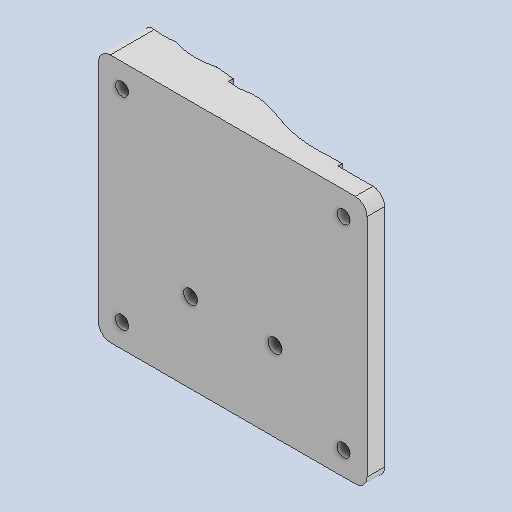
# Autodesk Inventor part: mouldingPlate_V6
Saved by Autodesk Inventor 2023 (Build 270158000, 158)
## iProperties
Created: 2023-03-15
Part Number: mouldingPlate_V6
Material: Generic
Document SubType Name: Modeling
Designer: shrey
Density: 1 g/cm^3
Appearance: Default
Author: shrey
Autodesk Inventor part; units mm, degrees
ref_plane "YZ Plane" through (0, 0, 0) normal (1, 0, 0) x (0, 1, 0)
ref_plane "XZ Plane" through (0, 0, 0) normal (0, 1, 0) x (-1, 0, 0)
ref_plane "XY Plane" through (0, 0, 0) normal (0, 0, 1) x (1, 0, 0)
ref_plane "Work Plane1" through (-64.2812, 0, 0) normal (0, 0, -1) x (1, 0, 0)
sketch "Sketch1" plane through (-64.2812, 0, 0) normal (0, 0, -1) x (1, 0, 0)
  line L0 (64.2812, -304.8) -> (64.2812, 304.8) construction
  line L1 (64.2812, -304.8) -> (0, -304.8) construction
  line L2 (6.11, 304.8) -> (0, 304.8) construction
  line L3 (0, -304.8) -> (6.11, -304.8) construction
  line L4 (6.2392, -19.8934) -> (64.0072, -19.8934) construction
  line L5 (64.0072, -19.8934) -> (64.0072, -14.3934) construction
  line L6 (64.0072, -14.3934) -> (6.2392, -14.3934) construction
  line L7 (6.2392, -14.3934) -> (6.2392, -19.8934) construction
  spline S0 degree 3 poles (60.7862, -9) (60.9061, -9.1901) (61.0858, -9.4753) (61.3069, -9.8666) (61.4657, -10.1639) (61.6162, -10.4656) (61.7579, -10.7714) (61.8899, -11.0816) (62.0114, -11.3961) (62.1204, -11.7151) (62.2163, -12.0383) (62.2788, -12.3122) (62.3239, -12.5324) (62.3716, -12.6943) (62.436, -12.8503) (62.5199, -12.997) (62.6084, -13.1066) (62.6883, -13.1859) (62.7558, -13.2363) (62.8251, -13.2847) (62.9013, -13.3209) (62.9789, -13.3544) (63.0609, -13.3742) (63.1437, -13.3909) (63.2562, -13.3949) (63.3966, -13.3923) (63.5369, -13.3949) (63.6495, -13.3909) (63.7322, -13.3742) (63.8143, -13.3544) (63.8918, -13.3209) (63.9681, -13.2847) (64.0373, -13.2363) (64.1049, -13.1859) (64.1848, -13.1066) (64.2733, -12.997) (64.3572, -12.8503) (64.4216, -12.6943) (64.4693, -12.5324) (64.5144, -12.3122) (64.5768, -12.0383) (64.6728, -11.7151) (64.7818, -11.3961) (64.9032, -11.0816) (65.0353, -10.7714) (65.177, -10.4656) (65.3275, -10.1639) (65.4863, -9.8666) (65.7074, -9.4753) (65.8871, -9.1901) (66.007, -9) knots 0 0 0 0 0.067405 0.101109 0.134814 0.168518 0.202222 0.235926 0.26963 0.303333 0.337035 0.370735 0.387584 0.40443 0.421277 0.438116 0.454951 0.463377 0.471802 0.480225 0.488651 0.497074 0.505499 0.513923 0.522347 0.5392 0.556053 0.564477 0.572901 0.581327 0.589749 0.598176 0.606598 0.615023 0.623449 0.640284 0.657123 0.67397 0.690816 0.707665 0.741365 0.775067 0.80877 0.842474 0.876178 0.909882 0.943586 0.977291 1.010995 1.0784 1.0784 1.0784 1.0784 construction
  line L8 (66.0072, -9) -> (66.007, -9) construction
  line L9 (66.0072, -20.8934) -> (66.0072, -9) construction
  line L10 (4.2392, -20.8934) -> (66.0072, -20.8934) construction
  line L11 (4.2392, -9) -> (4.2392, -20.8934) construction
  spline S1 degree 3 poles (4.2392, -9) (4.3591, -9.1901) (4.5388, -9.4753) (4.7599, -9.8666) (4.9187, -10.1639) (5.0692, -10.4656) (5.2109, -10.7714) (5.3429, -11.0816) (5.4644, -11.3961) (5.5734, -11.7151) (5.6693, -12.0383) (5.7318, -12.3122) (5.7769, -12.5324) (5.8246, -12.6943) (5.889, -12.8503) (5.9729, -12.997) (6.0614, -13.1066) (6.1413, -13.1859) (6.2088, -13.2363) (6.2781, -13.2847) (6.3543, -13.3209) (6.4319, -13.3544) (6.5139, -13.3742) (6.5967, -13.3909) (6.7092, -13.3949) (6.8496, -13.3923) (6.9899, -13.3949) (7.1025, -13.3909) (7.1852, -13.3742) (7.2673, -13.3544) (7.3448, -13.3209) (7.4211, -13.2847) (7.4903, -13.2363) (7.5579, -13.1859) (7.6378, -13.1066) (7.7263, -12.997) (7.8102, -12.8503) (7.8746, -12.6943) (7.9223, -12.5324) (7.9674, -12.3122) (8.0298, -12.0383) (8.1258, -11.7151) (8.2348, -11.3961) (8.3562, -11.0816) (8.4883, -10.7714) (8.63, -10.4656) (8.7805, -10.1639) (8.9393, -9.8666) (9.1604, -9.4753) (9.3401, -9.1901) (9.46, -9) knots 0 0 0 0 0.067405 0.101109 0.134814 0.168518 0.202222 0.235926 0.26963 0.303333 0.337035 0.370735 0.387584 0.40443 0.421277 0.438116 0.454951 0.463377 0.471802 0.480225 0.488651 0.497074 0.505499 0.513923 0.522347 0.5392 0.556053 0.564477 0.572901 0.581327 0.589749 0.598176 0.606598 0.615023 0.623449 0.640284 0.657123 0.67397 0.690816 0.707665 0.741365 0.775067 0.80877 0.842474 0.876178 0.909882 0.943586 0.977291 1.010995 1.0784 1.0784 1.0784 1.0784 construction
  line L12 (10.5222, -9) -> (9.46, -9) construction
  spline S2 degree 3 poles (10.5222, -9) (10.6421, -9.1901) (10.8218, -9.4753) (11.0429, -9.8666) (11.2017, -10.1639) (11.3522, -10.4656) (11.4939, -10.7714) (11.6259, -11.0816) (11.7474, -11.3961) (11.8564, -11.7151) (11.9523, -12.0383) (12.0148, -12.3122) (12.0599, -12.5324) (12.1076, -12.6943) (12.172, -12.8503) (12.2559, -12.997) (12.3444, -13.1066) (12.4243, -13.1859) (12.4918, -13.2363) (12.5611, -13.2847) (12.6373, -13.3209) (12.7149, -13.3544) (12.7969, -13.3742) (12.8797, -13.3909) (12.9922, -13.3949) (13.1326, -13.3923) (13.2729, -13.3949) (13.3855, -13.3909) (13.4682, -13.3742) (13.5503, -13.3544) (13.6278, -13.3209) (13.7041, -13.2847) (13.7733, -13.2363) (13.8409, -13.1859) (13.9208, -13.1066) (14.0093, -12.997) (14.0932, -12.8503) (14.1576, -12.6943) (14.2053, -12.5324) (14.2504, -12.3122) (14.3128, -12.0383) (14.4088, -11.7151) (14.5178, -11.3961) (14.6392, -11.0816) (14.7713, -10.7714) (14.913, -10.4656) (15.0635, -10.1639) (15.2223, -9.8666) (15.4434, -9.4753) (15.6231, -9.1901) (15.743, -9) knots 0 0 0 0 0.067405 0.101109 0.134814 0.168518 0.202222 0.235926 0.26963 0.303333 0.337035 0.370735 0.387584 0.40443 0.421277 0.438116 0.454951 0.463377 0.471802 0.480225 0.488651 0.497074 0.505499 0.513923 0.522347 0.5392 0.556053 0.564477 0.572901 0.581327 0.589749 0.598176 0.606598 0.615023 0.623449 0.640284 0.657123 0.67397 0.690816 0.707665 0.741365 0.775067 0.80877 0.842474 0.876178 0.909882 0.943586 0.977291 1.010995 1.0784 1.0784 1.0784 1.0784 construction
  line L13 (16.8052, -9) -> (15.743, -9) construction
  spline S3 degree 3 poles (16.8052, -9) (16.9251, -9.1901) (17.1048, -9.4753) (17.3259, -9.8666) (17.4847, -10.1639) (17.6352, -10.4656) (17.7769, -10.7714) (17.9089, -11.0816) (18.0304, -11.3961) (18.1394, -11.7151) (18.2353, -12.0383) (18.2978, -12.3122) (18.3429, -12.5324) (18.3906, -12.6943) (18.455, -12.8503) (18.5389, -12.997) (18.6274, -13.1066) (18.7073, -13.1859) (18.7748, -13.2363) (18.8441, -13.2847) (18.9203, -13.3209) (18.9979, -13.3544) (19.0799, -13.3742) (19.1627, -13.3909) (19.2752, -13.3949) (19.4156, -13.3923) (19.5559, -13.3949) (19.6685, -13.3909) (19.7512, -13.3742) (19.8333, -13.3544) (19.9108, -13.3209) (19.9871, -13.2847) (20.0563, -13.2363) (20.1239, -13.1859) (20.2038, -13.1066) (20.2923, -12.997) (20.3762, -12.8503) (20.4406, -12.6943) (20.4883, -12.5324) (20.5334, -12.3122) (20.5958, -12.0383) (20.6918, -11.7151) (20.8008, -11.3961) (20.9222, -11.0816) (21.0543, -10.7714) (21.196, -10.4656) (21.3465, -10.1639) (21.5053, -9.8666) (21.7264, -9.4753) (21.9061, -9.1901) (22.026, -9) knots 0 0 0 0 0.067405 0.101109 0.134814 0.168518 0.202222 0.235926 0.26963 0.303333 0.337035 0.370735 0.387584 0.40443 0.421277 0.438116 0.454951 0.463377 0.471802 0.480225 0.488651 0.497074 0.505499 0.513923 0.522347 0.5392 0.556053 0.564477 0.572901 0.581327 0.589749 0.598176 0.606598 0.615023 0.623449 0.640284 0.657123 0.67397 0.690816 0.707665 0.741365 0.775067 0.80877 0.842474 0.876178 0.909882 0.943586 0.977291 1.010995 1.0784 1.0784 1.0784 1.0784 construction
  line L14 (23.0882, -9) -> (22.026, -9) construction
  spline S4 degree 3 poles (23.0882, -9) (23.2081, -9.1901) (23.3878, -9.4753) (23.6089, -9.8666) (23.7677, -10.1639) (23.9182, -10.4656) (24.0599, -10.7714) (24.1919, -11.0816) (24.3134, -11.3961) (24.4224, -11.7151) (24.5183, -12.0383) (24.5808, -12.3122) (24.6259, -12.5324) (24.6736, -12.6943) (24.738, -12.8503) (24.8219, -12.997) (24.9104, -13.1066) (24.9903, -13.1859) (25.0578, -13.2363) (25.1271, -13.2847) (25.2033, -13.3209) (25.2809, -13.3544) (25.3629, -13.3742) (25.4457, -13.3909) (25.5582, -13.3949) (25.6986, -13.3923) (25.8389, -13.3949) (25.9515, -13.3909) (26.0342, -13.3742) (26.1163, -13.3544) (26.1938, -13.3209) (26.2701, -13.2847) (26.3393, -13.2363) (26.4069, -13.1859) (26.4868, -13.1066) (26.5753, -12.997) (26.6592, -12.8503) (26.7236, -12.6943) (26.7713, -12.5324) (26.8164, -12.3122) (26.8788, -12.0383) (26.9748, -11.7151) (27.0838, -11.3961) (27.2052, -11.0816) (27.3373, -10.7714) (27.479, -10.4656) (27.6295, -10.1639) (27.7883, -9.8666) (28.0094, -9.4753) (28.1891, -9.1901) (28.309, -9) knots 0 0 0 0 0.067405 0.101109 0.134814 0.168518 0.202222 0.235926 0.26963 0.303333 0.337035 0.370735 0.387584 0.40443 0.421277 0.438116 0.454951 0.463377 0.471802 0.480225 0.488651 0.497074 0.505499 0.513923 0.522347 0.5392 0.556053 0.564477 0.572901 0.581327 0.589749 0.598176 0.606598 0.615023 0.623449 0.640284 0.657123 0.67397 0.690816 0.707665 0.741365 0.775067 0.80877 0.842474 0.876178 0.909882 0.943586 0.977291 1.010995 1.0784 1.0784 1.0784 1.0784 construction
  line L15 (29.3712, -9) -> (28.309, -9) construction
  spline S5 degree 3 poles (29.3712, -9) (29.4911, -9.1901) (29.6708, -9.4753) (29.8919, -9.8666) (30.0507, -10.1639) (30.2012, -10.4656) (30.3429, -10.7714) (30.4749, -11.0816) (30.5964, -11.3961) (30.7054, -11.7151) (30.8013, -12.0383) (30.8638, -12.3122) (30.9089, -12.5324) (30.9566, -12.6943) (31.021, -12.8503) (31.1049, -12.997) (31.1934, -13.1066) (31.2733, -13.1859) (31.3408, -13.2363) (31.4101, -13.2847) (31.4863, -13.3209) (31.5639, -13.3544) (31.6459, -13.3742) (31.7287, -13.3909) (31.8412, -13.3949) (31.9816, -13.3923) (32.1219, -13.3949) (32.2345, -13.3909) (32.3172, -13.3742) (32.3993, -13.3544) (32.4768, -13.3209) (32.5531, -13.2847) (32.6223, -13.2363) (32.6899, -13.1859) (32.7698, -13.1066) (32.8583, -12.997) (32.9422, -12.8503) (33.0066, -12.6943) (33.0543, -12.5324) (33.0994, -12.3122) (33.1618, -12.0383) (33.2578, -11.7151) (33.3668, -11.3961) (33.4882, -11.0816) (33.6203, -10.7714) (33.762, -10.4656) (33.9125, -10.1639) (34.0713, -9.8666) (34.2924, -9.4753) (34.4721, -9.1901) (34.592, -9) knots 0 0 0 0 0.067405 0.101109 0.134814 0.168518 0.202222 0.235926 0.26963 0.303333 0.337035 0.370735 0.387584 0.40443 0.421277 0.438116 0.454951 0.463377 0.471802 0.480225 0.488651 0.497074 0.505499 0.513923 0.522347 0.5392 0.556053 0.564477 0.572901 0.581327 0.589749 0.598176 0.606598 0.615023 0.623449 0.640284 0.657123 0.67397 0.690816 0.707665 0.741365 0.775067 0.80877 0.842474 0.876178 0.909882 0.943586 0.977291 1.010995 1.0784 1.0784 1.0784 1.0784 construction
  line L16 (35.6542, -9) -> (34.592, -9) construction
  spline S6 degree 3 poles (35.6542, -9) (35.7741, -9.1901) (35.9538, -9.4753) (36.1749, -9.8666) (36.3337, -10.1639) (36.4842, -10.4656) (36.6259, -10.7714) (36.7579, -11.0816) (36.8794, -11.3961) (36.9884, -11.7151) (37.0843, -12.0383) (37.1468, -12.3122) (37.1919, -12.5324) (37.2396, -12.6943) (37.304, -12.8503) (37.3879, -12.997) (37.4764, -13.1066) (37.5563, -13.1859) (37.6238, -13.2363) (37.6931, -13.2847) (37.7693, -13.3209) (37.8469, -13.3544) (37.9289, -13.3742) (38.0117, -13.3909) (38.1242, -13.3949) (38.2646, -13.3923) (38.4049, -13.3949) (38.5175, -13.3909) (38.6002, -13.3742) (38.6823, -13.3544) (38.7598, -13.3209) (38.8361, -13.2847) (38.9053, -13.2363) (38.9729, -13.1859) (39.0528, -13.1066) (39.1413, -12.997) (39.2252, -12.8503) (39.2896, -12.6943) (39.3373, -12.5324) (39.3824, -12.3122) (39.4448, -12.0383) (39.5408, -11.7151) (39.6498, -11.3961) (39.7712, -11.0816) (39.9033, -10.7714) (40.045, -10.4656) (40.1955, -10.1639) (40.3543, -9.8666) (40.5754, -9.4753) (40.7551, -9.1901) (40.875, -9) knots 0 0 0 0 0.067405 0.101109 0.134814 0.168518 0.202222 0.235926 0.26963 0.303333 0.337035 0.370735 0.387584 0.40443 0.421277 0.438116 0.454951 0.463377 0.471802 0.480225 0.488651 0.497074 0.505499 0.513923 0.522347 0.5392 0.556053 0.564477 0.572901 0.581327 0.589749 0.598176 0.606598 0.615023 0.623449 0.640284 0.657123 0.67397 0.690816 0.707665 0.741365 0.775067 0.80877 0.842474 0.876178 0.909882 0.943586 0.977291 1.010995 1.0784 1.0784 1.0784 1.0784 construction
  line L17 (41.9372, -9) -> (40.875, -9) construction
  spline S7 degree 3 poles (41.9372, -9) (42.0571, -9.1901) (42.2368, -9.4753) (42.4579, -9.8666) (42.6167, -10.1639) (42.7672, -10.4656) (42.9089, -10.7714) (43.0409, -11.0816) (43.1624, -11.3961) (43.2714, -11.7151) (43.3673, -12.0383) (43.4298, -12.3122) (43.4749, -12.5324) (43.5226, -12.6943) (43.587, -12.8503) (43.6709, -12.997) (43.7594, -13.1066) (43.8393, -13.1859) (43.9068, -13.2363) (43.9761, -13.2847) (44.0523, -13.3209) (44.1299, -13.3544) (44.2119, -13.3742) (44.2947, -13.3909) (44.4072, -13.3949) (44.5476, -13.3923) (44.6879, -13.3949) (44.8005, -13.3909) (44.8832, -13.3742) (44.9653, -13.3544) (45.0428, -13.3209) (45.1191, -13.2847) (45.1883, -13.2363) (45.2559, -13.1859) (45.3358, -13.1066) (45.4243, -12.997) (45.5082, -12.8503) (45.5726, -12.6943) (45.6203, -12.5324) (45.6654, -12.3122) (45.7278, -12.0383) (45.8238, -11.7151) (45.9328, -11.3961) (46.0542, -11.0816) (46.1863, -10.7714) (46.328, -10.4656) (46.4785, -10.1639) (46.6373, -9.8666) (46.8584, -9.4753) (47.0381, -9.1901) (47.158, -9) knots 0 0 0 0 0.067405 0.101109 0.134814 0.168518 0.202222 0.235926 0.26963 0.303333 0.337035 0.370735 0.387584 0.40443 0.421277 0.438116 0.454951 0.463377 0.471802 0.480225 0.488651 0.497074 0.505499 0.513923 0.522347 0.5392 0.556053 0.564477 0.572901 0.581327 0.589749 0.598176 0.606598 0.615023 0.623449 0.640284 0.657123 0.67397 0.690816 0.707665 0.741365 0.775067 0.80877 0.842474 0.876178 0.909882 0.943586 0.977291 1.010995 1.0784 1.0784 1.0784 1.0784 construction
  line L18 (48.2202, -9) -> (47.158, -9) construction
  spline S8 degree 3 poles (48.2202, -9) (48.3401, -9.1901) (48.5198, -9.4753) (48.7409, -9.8666) (48.8997, -10.1639) (49.0502, -10.4656) (49.1919, -10.7714) (49.3239, -11.0816) (49.4454, -11.3961) (49.5544, -11.7151) (49.6503, -12.0383) (49.7128, -12.3122) (49.7579, -12.5324) (49.8056, -12.6943) (49.87, -12.8503) (49.9539, -12.997) (50.0424, -13.1066) (50.1223, -13.1859) (50.1898, -13.2363) (50.2591, -13.2847) (50.3353, -13.3209) (50.4129, -13.3544) (50.4949, -13.3742) (50.5777, -13.3909) (50.6902, -13.3949) (50.8306, -13.3923) (50.9709, -13.3949) (51.0835, -13.3909) (51.1662, -13.3742) (51.2483, -13.3544) (51.3258, -13.3209) (51.4021, -13.2847) (51.4713, -13.2363) (51.5389, -13.1859) (51.6188, -13.1066) (51.7073, -12.997) (51.7912, -12.8503) (51.8556, -12.6943) (51.9033, -12.5324) (51.9484, -12.3122) (52.0108, -12.0383) (52.1068, -11.7151) (52.2158, -11.3961) (52.3372, -11.0816) (52.4693, -10.7714) (52.611, -10.4656) (52.7615, -10.1639) (52.9203, -9.8666) (53.1414, -9.4753) (53.3211, -9.1901) (53.441, -9) knots 0 0 0 0 0.067405 0.101109 0.134814 0.168518 0.202222 0.235926 0.26963 0.303333 0.337035 0.370735 0.387584 0.40443 0.421277 0.438116 0.454951 0.463377 0.471802 0.480225 0.488651 0.497074 0.505499 0.513923 0.522347 0.5392 0.556053 0.564477 0.572901 0.581327 0.589749 0.598176 0.606598 0.615023 0.623449 0.640284 0.657123 0.67397 0.690816 0.707665 0.741365 0.775067 0.80877 0.842474 0.876178 0.909882 0.943586 0.977291 1.010995 1.0784 1.0784 1.0784 1.0784 construction
  line L19 (54.5032, -9) -> (53.441, -9) construction
  spline S9 degree 3 poles (54.5032, -9) (54.6231, -9.1901) (54.8028, -9.4753) (55.0239, -9.8666) (55.1827, -10.1639) (55.3332, -10.4656) (55.4749, -10.7714) (55.6069, -11.0816) (55.7284, -11.3961) (55.8374, -11.7151) (55.9333, -12.0383) (55.9958, -12.3122) (56.0409, -12.5324) (56.0886, -12.6943) (56.153, -12.8503) (56.2369, -12.997) (56.3254, -13.1066) (56.4053, -13.1859) (56.4728, -13.2363) (56.5421, -13.2847) (56.6183, -13.3209) (56.6959, -13.3544) (56.7779, -13.3742) (56.8607, -13.3909) (56.9732, -13.3949) (57.1136, -13.3923) (57.2539, -13.3949) (57.3665, -13.3909) (57.4492, -13.3742) (57.5313, -13.3544) (57.6088, -13.3209) (57.6851, -13.2847) (57.7543, -13.2363) (57.8219, -13.1859) (57.9018, -13.1066) (57.9903, -12.997) (58.0742, -12.8503) (58.1386, -12.6943) (58.1863, -12.5324) (58.2314, -12.3122) (58.2938, -12.0383) (58.3898, -11.7151) (58.4988, -11.3961) (58.6202, -11.0816) (58.7523, -10.7714) (58.894, -10.4656) (59.0445, -10.1639) (59.2033, -9.8666) (59.4244, -9.4753) (59.6041, -9.1901) (59.724, -9) knots 0 0 0 0 0.067405 0.101109 0.134814 0.168518 0.202222 0.235926 0.26963 0.303333 0.337035 0.370735 0.387584 0.40443 0.421277 0.438116 0.454951 0.463377 0.471802 0.480225 0.488651 0.497074 0.505499 0.513923 0.522347 0.5392 0.556053 0.564477 0.572901 0.581327 0.589749 0.598176 0.606598 0.615023 0.623449 0.640284 0.657123 0.67397 0.690816 0.707665 0.741365 0.775067 0.80877 0.842474 0.876178 0.909882 0.943586 0.977291 1.010995 1.0784 1.0784 1.0784 1.0784 construction
  line L20 (60.7862, -9) -> (59.724, -9) construction
  arc A0 (16.2895, -1.1) -> (21.5957, -6.4062) centre (22.6957, 0) ccw construction
  line L21 (21.5957, -6.4062) -> (21.5957, -2.8983) construction
  arc A1 (19.7974, -1.1) -> (21.5957, -2.8983) centre (22.6957, 0) ccw construction
  line L22 (19.7974, -1.1) -> (16.2895, -1.1) construction
  arc A2 (21.5957, 6.4062) -> (16.2895, 1.1) centre (22.6957, 0) ccw construction
  line L23 (16.2895, 1.1) -> (19.7974, 1.1) construction
  arc A3 (21.5957, 2.8983) -> (19.7974, 1.1) centre (22.6957, 0) ccw construction
  line L24 (21.5957, 2.8983) -> (21.5957, 6.4062) construction
  line L25 (23.7957, -2.8983) -> (23.7957, -6.4062) construction
  arc A4 (23.7957, -6.4062) -> (29.102, -1.1) centre (22.6957, 0) ccw construction
  line L26 (29.102, -1.1) -> (25.594, -1.1) construction
  arc A5 (23.7957, -2.8983) -> (25.594, -1.1) centre (22.6957, 0) ccw construction
  arc A6 (29.102, 1.1) -> (23.7957, 6.4062) centre (22.6957, 0) ccw construction
  line L27 (23.7957, 6.4062) -> (23.7957, 2.8983) construction
  arc A7 (25.594, 1.1) -> (23.7957, 2.8983) centre (22.6957, 0) ccw construction
  line L28 (25.594, 1.1) -> (29.102, 1.1) construction
  circle A8 centre (22.6957, 0) radius 1.1 construction
  spline S10 degree 3 poles (18.2825, -8.3602) (18.3162, -8.3172) (18.3835, -8.2311) (18.4765, -8.0961) (18.562, -7.9561) (18.6361, -7.8099) (18.7049, -7.6609) (18.7574, -7.5055) (18.7991, -7.3469) (18.8247, -7.1847) (18.8317, -7.0206) (18.8197, -6.8568) (18.7857, -6.696) (18.7274, -6.5424) (18.6479, -6.3984) (18.5617, -6.2919) (18.4849, -6.214) (18.3987, -6.1466) (18.2867, -6.0685) (18.1778, -5.9861) (18.087, -5.925) (17.9892, -5.876) (17.8613, -5.8269) (17.6998, -5.7958) (17.5357, -5.7878) (17.3723, -5.8052) (17.2128, -5.8443) (17.0589, -5.9017) (16.9125, -5.9762) (16.7746, -6.0649) (16.643, -6.1629) (16.5226, -6.2743) (16.4064, -6.39) (16.2997, -6.5145) (16.2, -6.6448) (16.139, -6.7354) (16.1084, -6.7807) knots -0.524268 -0.524268 -0.524268 -0.524268 -0.507879 -0.49149 -0.475102 -0.458716 -0.44233 -0.425942 -0.409559 -0.393171 -0.376784 -0.360403 -0.344025 -0.327651 -0.311278 -0.294912 -0.286715 -0.278522 -0.262134 -0.245745 -0.237552 -0.229355 -0.21299 -0.196616 -0.180243 -0.163864 -0.147483 -0.131097 -0.114709 -0.098325 -0.081938 -0.065552 -0.049165 -0.032777 -0.016389 0 0 0 0 construction
  spline S11 degree 3 poles (16.1084, -6.7807) (16.0601, -6.8172) (15.9634, -6.8903) (15.806, -6.9815) (15.6442, -7.0641) (15.4224, -7.1618) (15.1372, -7.2645) (14.7865, -7.3605) (14.4302, -7.4327) (14.0701, -7.4825) (13.7079, -7.5136) (13.4657, -7.5181) (13.3446, -7.5204) knots 0 0 0 0 0.062477 0.124976 0.18748 0.249986 0.374973 0.499971 0.624974 0.749982 0.874991 1 1 1 1 construction
  arc A9 (12.6538, -6.5696) -> (13.3446, -7.5204) centre (22.6957, 0) ccw construction
  spline S12 degree 3 poles (12.6538, -6.5696) (12.6933, -6.4551) (12.7725, -6.2261) (12.914, -5.8912) (13.0726, -5.5642) (13.2514, -5.2476) (13.4511, -4.9437) (13.6368, -4.7042) (13.7983, -4.5235) (13.9268, -4.3951) (14.0623, -4.2736) (14.1616, -4.2042) (14.2113, -4.1695) knots 0 0 0 0 0.125009 0.250018 0.375026 0.500029 0.625027 0.750014 0.81252 0.875024 0.937523 1 1 1 1 construction
  spline S13 degree 3 poles (14.2113, -4.1695) (14.2639, -4.1545) (14.3689, -4.1244) (14.5235, -4.0699) (14.675, -4.0069) (14.8209, -3.9321) (14.9641, -3.8521) (15.0979, -3.7572) (15.2249, -3.6534) (15.341, -3.5372) (15.4431, -3.4086) (15.5296, -3.269) (15.5967, -3.1189) (15.6398, -2.9603) (15.6601, -2.7972) (15.6529, -2.6603) (15.6366, -2.5522) (15.6065, -2.447) (15.5618, -2.318) (15.5222, -2.1873) (15.4846, -2.0845) (15.4342, -1.9874) (15.3596, -1.8725) (15.2473, -1.7524) (15.1192, -1.6495) (14.9767, -1.5675) (14.8247, -1.5054) (14.6665, -1.4613) (14.5043, -1.4356) (14.3406, -1.4263) (14.1765, -1.4282) (14.0136, -1.4475) (13.8516, -1.4728) (13.6921, -1.5109) (13.5349, -1.5576) (13.4322, -1.5951) (13.3809, -1.6138) knots -0.524268 -0.524268 -0.524268 -0.524268 -0.507879 -0.49149 -0.475102 -0.458716 -0.44233 -0.425942 -0.409559 -0.393171 -0.376784 -0.360403 -0.344025 -0.327651 -0.311278 -0.294912 -0.286715 -0.278522 -0.262134 -0.245745 -0.237552 -0.229355 -0.21299 -0.196616 -0.180243 -0.163864 -0.147483 -0.131097 -0.114709 -0.098325 -0.081938 -0.065552 -0.049165 -0.032777 -0.016389 0 0 0 0 construction
  spline S14 degree 3 poles (13.3809, -1.6138) (13.3203, -1.6149) (13.1992, -1.6172) (13.0182, -1.5985) (12.8387, -1.5702) (12.6019, -1.5189) (12.3108, -1.4343) (11.9706, -1.3059) (11.64, -1.1548) (11.3194, -0.9835) (11.0081, -0.7957) (10.8094, -0.657) (10.7101, -0.5876) knots 0 0 0 0 0.062477 0.124976 0.18748 0.249986 0.374973 0.499971 0.624974 0.749982 0.874991 1 1 1 1 construction
  arc A10 (10.7101, 0.5876) -> (10.7101, -0.5876) centre (22.6957, 0) ccw construction
  spline S15 degree 3 poles (10.7101, 0.5876) (10.8094, 0.657) (11.0081, 0.7957) (11.3194, 0.9835) (11.64, 1.1548) (11.9706, 1.3059) (12.3108, 1.4343) (12.6019, 1.5189) (12.8387, 1.5702) (13.0182, 1.5985) (13.1992, 1.6172) (13.3203, 1.6149) (13.3809, 1.6138) knots 0 0 0 0 0.125009 0.250018 0.375026 0.500029 0.625027 0.750014 0.81252 0.875024 0.937523 1 1 1 1 construction
  spline S16 degree 3 poles (13.3809, 1.6138) (13.4322, 1.5951) (13.5349, 1.5576) (13.6921, 1.5109) (13.8516, 1.4728) (14.0136, 1.4475) (14.1765, 1.4282) (14.3406, 1.4263) (14.5043, 1.4356) (14.6665, 1.4613) (14.8247, 1.5054) (14.9767, 1.5675) (15.1192, 1.6495) (15.2473, 1.7524) (15.3596, 1.8725) (15.4342, 1.9874) (15.4846, 2.0845) (15.5222, 2.1873) (15.5618, 2.318) (15.6065, 2.447) (15.6366, 2.5522) (15.6529, 2.6603) (15.6601, 2.7972) (15.6398, 2.9603) (15.5967, 3.1189) (15.5296, 3.269) (15.4431, 3.4086) (15.341, 3.5372) (15.2249, 3.6534) (15.0979, 3.7572) (14.9641, 3.8521) (14.8209, 3.9321) (14.675, 4.0069) (14.5235, 4.0699) (14.3689, 4.1244) (14.2639, 4.1545) (14.2113, 4.1695) knots -0.524268 -0.524268 -0.524268 -0.524268 -0.507879 -0.49149 -0.475102 -0.458716 -0.44233 -0.425942 -0.409559 -0.393171 -0.376784 -0.360403 -0.344025 -0.327651 -0.311278 -0.294912 -0.286715 -0.278522 -0.262134 -0.245745 -0.237552 -0.229355 -0.21299 -0.196616 -0.180243 -0.163864 -0.147483 -0.131097 -0.114709 -0.098325 -0.081938 -0.065552 -0.049165 -0.032777 -0.016389 0 0 0 0 construction
  spline S17 degree 3 poles (14.2113, 4.1695) (14.1616, 4.2042) (14.0623, 4.2736) (13.9268, 4.3951) (13.7983, 4.5235) (13.6368, 4.7042) (13.4511, 4.9437) (13.2514, 5.2476) (13.0726, 5.5642) (12.914, 5.8912) (12.7725, 6.2261) (12.6933, 6.4551) (12.6538, 6.5696) knots 0 0 0 0 0.062477 0.124976 0.18748 0.249986 0.374973 0.499971 0.624974 0.749982 0.874991 1 1 1 1 construction
  arc A11 (13.3446, 7.5204) -> (12.6538, 6.5696) centre (22.6957, 0) ccw construction
  spline S18 degree 3 poles (13.3446, 7.5204) (13.4657, 7.5181) (13.7079, 7.5136) (14.0701, 7.4825) (14.4302, 7.4327) (14.7865, 7.3605) (15.1372, 7.2645) (15.4224, 7.1618) (15.6442, 7.0641) (15.806, 6.9815) (15.9634, 6.8903) (16.0601, 6.8172) (16.1084, 6.7807) knots 0 0 0 0 0.125009 0.250018 0.375026 0.500029 0.625027 0.750014 0.81252 0.875024 0.937523 1 1 1 1 construction
  spline S19 degree 3 poles (16.1084, 6.7807) (16.139, 6.7354) (16.2, 6.6448) (16.2997, 6.5145) (16.4064, 6.39) (16.5226, 6.2743) (16.643, 6.1629) (16.7746, 6.0649) (16.9125, 5.9762) (17.0589, 5.9017) (17.2128, 5.8443) (17.3723, 5.8052) (17.5357, 5.7878) (17.6998, 5.7958) (17.8613, 5.8269) (17.9892, 5.876) (18.087, 5.925) (18.1778, 5.9861) (18.2867, 6.0685) (18.3987, 6.1466) (18.4849, 6.214) (18.5617, 6.2919) (18.6479, 6.3984) (18.7274, 6.5424) (18.7857, 6.696) (18.8197, 6.8568) (18.8317, 7.0206) (18.8247, 7.1847) (18.7991, 7.3469) (18.7574, 7.5055) (18.7049, 7.6609) (18.6361, 7.8099) (18.562, 7.9561) (18.4765, 8.0961) (18.3835, 8.2311) (18.3162, 8.3172) (18.2825, 8.3602) knots -0.524268 -0.524268 -0.524268 -0.524268 -0.507879 -0.49149 -0.475102 -0.458716 -0.44233 -0.425942 -0.409559 -0.393171 -0.376784 -0.360403 -0.344025 -0.327651 -0.311278 -0.294912 -0.286715 -0.278522 -0.262134 -0.245745 -0.237552 -0.229355 -0.21299 -0.196616 -0.180243 -0.163864 -0.147483 -0.131097 -0.114709 -0.098325 -0.081938 -0.065552 -0.049165 -0.032777 -0.016389 0 0 0 0 construction
  spline S20 degree 3 poles (18.2825, 8.3602) (18.2627, 8.4175) (18.2231, 8.532) (18.1849, 8.7099) (18.1564, 8.8894) (18.132, 9.1304) (18.1225, 9.4334) (18.1395, 9.7966) (18.181, 10.1578) (18.2449, 10.5156) (18.3273, 10.8697) (18.3978, 11.1015) (18.4331, 11.2174) knots 0 0 0 0 0.062477 0.124976 0.18748 0.249986 0.374973 0.499971 0.624974 0.749982 0.874991 1 1 1 1 construction
  arc A12 (19.5508, 11.5806) -> (18.4331, 11.2174) centre (22.6957, 0) ccw construction
  spline S21 degree 3 poles (19.5508, 11.5806) (19.6475, 11.5076) (19.8408, 11.3615) (20.1156, 11.1235) (20.3776, 10.8715) (20.6235, 10.6037) (20.8507, 10.3199) (21.0211, 10.0692) (21.143, 9.8598) (21.2255, 9.6979) (21.2992, 9.5315) (21.3344, 9.4156) (21.3521, 9.3576) knots 0 0 0 0 0.125009 0.250018 0.375026 0.500029 0.625027 0.750014 0.81252 0.875024 0.937523 1 1 1 1 construction
  spline S22 degree 3 poles (21.3521, 9.3576) (21.3501, 9.303) (21.3463, 9.1938) (21.3504, 9.0299) (21.3635, 8.8664) (21.3895, 8.7045) (21.4214, 8.5436) (21.4703, 8.3869) (21.5297, 8.2341) (21.6044, 8.0878) (21.6951, 7.951) (21.8012, 7.8256) (21.9232, 7.7154) (22.0607, 7.6254) (22.2096, 7.5557) (22.3419, 7.5202) (22.4498, 7.5023) (22.5592, 7.4984) (22.6957, 7.5011) (22.8322, 7.4984) (22.9416, 7.5023) (23.0495, 7.5202) (23.1818, 7.5557) (23.3308, 7.6254) (23.4682, 7.7154) (23.5903, 7.8256) (23.6963, 7.951) (23.7871, 8.0878) (23.8617, 8.2341) (23.9211, 8.3869) (23.97, 8.5436) (24.002, 8.7045) (24.028, 8.8664) (24.041, 9.0299) (24.0451, 9.1938) (24.0413, 9.303) (24.0394, 9.3576) knots -0.524268 -0.524268 -0.524268 -0.524268 -0.507879 -0.49149 -0.475102 -0.458716 -0.44233 -0.425942 -0.409559 -0.393171 -0.376784 -0.360403 -0.344025 -0.327651 -0.311278 -0.294912 -0.286715 -0.278522 -0.262134 -0.245745 -0.237552 -0.229355 -0.21299 -0.196616 -0.180243 -0.163864 -0.147483 -0.131097 -0.114709 -0.098325 -0.081938 -0.065552 -0.049165 -0.032777 -0.016389 0 0 0 0 construction
  spline S23 degree 3 poles (24.0394, 9.3576) (24.057, 9.4156) (24.0923, 9.5315) (24.166, 9.6979) (24.2484, 9.8598) (24.3703, 10.0692) (24.5407, 10.3199) (24.768, 10.6037) (25.0139, 10.8715) (25.2758, 11.1235) (25.5507, 11.3615) (25.744, 11.5076) (25.8406, 11.5806) knots 0 0 0 0 0.062477 0.124976 0.18748 0.249986 0.374973 0.499971 0.624974 0.749982 0.874991 1 1 1 1 construction
  arc A13 (26.9583, 11.2174) -> (25.8406, 11.5806) centre (22.6957, 0) ccw construction
  spline S24 degree 3 poles (26.9583, 11.2174) (26.9936, 11.1015) (27.0642, 10.8697) (27.1466, 10.5156) (27.2104, 10.1578) (27.2519, 9.7966) (27.2689, 9.4334) (27.2594, 9.1304) (27.235, 8.8894) (27.2065, 8.7099) (27.1684, 8.532) (27.1287, 8.4175) (27.1089, 8.3602) knots 0 0 0 0 0.125009 0.250018 0.375026 0.500029 0.625027 0.750014 0.81252 0.875024 0.937523 1 1 1 1 construction
  spline S25 degree 3 poles (27.1089, 8.3602) (27.0753, 8.3172) (27.008, 8.2311) (26.9149, 8.0961) (26.8294, 7.9561) (26.7553, 7.8099) (26.6866, 7.6609) (26.6341, 7.5055) (26.5923, 7.3469) (26.5667, 7.1847) (26.5597, 7.0206) (26.5718, 6.8568) (26.6057, 6.696) (26.6641, 6.5424) (26.7436, 6.3984) (26.8298, 6.2919) (26.9065, 6.214) (26.9927, 6.1466) (27.1047, 6.0685) (27.2136, 5.9861) (27.3044, 5.925) (27.4022, 5.876) (27.5301, 5.8269) (27.6916, 5.7958) (27.8557, 5.7878) (28.0192, 5.8052) (28.1787, 5.8443) (28.3325, 5.9017) (28.4789, 5.9762) (28.6168, 6.0649) (28.7485, 6.1629) (28.8689, 6.2743) (28.985, 6.39) (29.0917, 6.5145) (29.1914, 6.6448) (29.2525, 6.7354) (29.283, 6.7807) knots -0.524268 -0.524268 -0.524268 -0.524268 -0.507879 -0.49149 -0.475102 -0.458716 -0.44233 -0.425942 -0.409559 -0.393171 -0.376784 -0.360403 -0.344025 -0.327651 -0.311278 -0.294912 -0.286715 -0.278522 -0.262134 -0.245745 -0.237552 -0.229355 -0.21299 -0.196616 -0.180243 -0.163864 -0.147483 -0.131097 -0.114709 -0.098325 -0.081938 -0.065552 -0.049165 -0.032777 -0.016389 0 0 0 0 construction
  spline S26 degree 3 poles (29.283, 6.7807) (29.3313, 6.8172) (29.428, 6.8903) (29.5854, 6.9815) (29.7473, 7.0641) (29.969, 7.1618) (30.2542, 7.2645) (30.6049, 7.3605) (30.9612, 7.4327) (31.3213, 7.4825) (31.6835, 7.5136) (31.9258, 7.5181) (32.0469, 7.5204) knots 0 0 0 0 0.062477 0.124976 0.18748 0.249986 0.374973 0.499971 0.624974 0.749982 0.874991 1 1 1 1 construction
  arc A14 (32.7377, 6.5696) -> (32.0469, 7.5204) centre (22.6957, 0) ccw construction
  spline S27 degree 3 poles (32.7377, 6.5696) (32.6981, 6.4551) (32.6189, 6.2261) (32.4775, 5.8912) (32.3188, 5.5642) (32.1401, 5.2476) (31.9403, 4.9437) (31.7546, 4.7042) (31.5931, 4.5235) (31.4646, 4.3951) (31.3292, 4.2736) (31.2298, 4.2042) (31.1801, 4.1695) knots 0 0 0 0 0.125009 0.250018 0.375026 0.500029 0.625027 0.750014 0.81252 0.875024 0.937523 1 1 1 1 construction
  spline S28 degree 3 poles (31.1801, 4.1695) (31.1276, 4.1545) (31.0225, 4.1244) (30.8679, 4.0699) (30.7164, 4.0069) (30.5705, 3.9321) (30.4274, 3.8521) (30.2935, 3.7572) (30.1665, 3.6534) (30.0504, 3.5372) (29.9483, 3.4086) (29.8618, 3.269) (29.7948, 3.1189) (29.7517, 2.9603) (29.7314, 2.7972) (29.7386, 2.6603) (29.7549, 2.5522) (29.7849, 2.447) (29.8297, 2.318) (29.8693, 2.1873) (29.9068, 2.0845) (29.9572, 1.9874) (30.0318, 1.8725) (30.1442, 1.7524) (30.2722, 1.6495) (30.4147, 1.5675) (30.5667, 1.5054) (30.7249, 1.4613) (30.8871, 1.4356) (31.0509, 1.4263) (31.2149, 1.4282) (31.3778, 1.4475) (31.5398, 1.4728) (31.6994, 1.5109) (31.8565, 1.5576) (31.9592, 1.5951) (32.0105, 1.6138) knots -0.524268 -0.524268 -0.524268 -0.524268 -0.507879 -0.49149 -0.475102 -0.458716 -0.44233 -0.425942 -0.409559 -0.393171 -0.376784 -0.360403 -0.344025 -0.327651 -0.311278 -0.294912 -0.286715 -0.278522 -0.262134 -0.245745 -0.237552 -0.229355 -0.21299 -0.196616 -0.180243 -0.163864 -0.147483 -0.131097 -0.114709 -0.098325 -0.081938 -0.065552 -0.049165 -0.032777 -0.016389 0 0 0 0 construction
  spline S29 degree 3 poles (32.0105, 1.6138) (32.0711, 1.6149) (32.1923, 1.6172) (32.3733, 1.5985) (32.5527, 1.5702) (32.7896, 1.5189) (33.0806, 1.4343) (33.4208, 1.3059) (33.7515, 1.1548) (34.0721, 0.9835) (34.3834, 0.7957) (34.582, 0.657) (34.6813, 0.5876) knots 0 0 0 0 0.062477 0.124976 0.18748 0.249986 0.374973 0.499971 0.624974 0.749982 0.874991 1 1 1 1 construction
  arc A15 (34.6813, -0.5876) -> (34.6813, 0.5876) centre (22.6957, 0) ccw construction
  spline S30 degree 3 poles (34.6813, -0.5876) (34.582, -0.657) (34.3834, -0.7957) (34.0721, -0.9835) (33.7515, -1.1548) (33.4208, -1.3059) (33.0806, -1.4343) (32.7896, -1.5189) (32.5527, -1.5702) (32.3733, -1.5985) (32.1923, -1.6172) (32.0711, -1.6149) (32.0105, -1.6138) knots 0 0 0 0 0.125009 0.250018 0.375026 0.500029 0.625027 0.750014 0.81252 0.875024 0.937523 1 1 1 1 construction
  spline S31 degree 3 poles (32.0105, -1.6138) (31.9592, -1.5951) (31.8565, -1.5576) (31.6994, -1.5109) (31.5398, -1.4728) (31.3778, -1.4475) (31.2149, -1.4282) (31.0509, -1.4263) (30.8871, -1.4356) (30.7249, -1.4613) (30.5667, -1.5054) (30.4147, -1.5675) (30.2722, -1.6495) (30.1442, -1.7524) (30.0318, -1.8725) (29.9572, -1.9874) (29.9068, -2.0845) (29.8693, -2.1873) (29.8297, -2.318) (29.7849, -2.447) (29.7549, -2.5522) (29.7386, -2.6603) (29.7314, -2.7972) (29.7517, -2.9603) (29.7948, -3.1189) (29.8618, -3.269) (29.9483, -3.4086) (30.0504, -3.5372) (30.1665, -3.6534) (30.2935, -3.7572) (30.4274, -3.8521) (30.5705, -3.9321) (30.7164, -4.0069) (30.8679, -4.0699) (31.0225, -4.1244) (31.1276, -4.1545) (31.1801, -4.1695) knots -0.524268 -0.524268 -0.524268 -0.524268 -0.507879 -0.49149 -0.475102 -0.458716 -0.44233 -0.425942 -0.409559 -0.393171 -0.376784 -0.360403 -0.344025 -0.327651 -0.311278 -0.294912 -0.286715 -0.278522 -0.262134 -0.245745 -0.237552 -0.229355 -0.21299 -0.196616 -0.180243 -0.163864 -0.147483 -0.131097 -0.114709 -0.098325 -0.081938 -0.065552 -0.049165 -0.032777 -0.016389 0 0 0 0 construction
  spline S32 degree 3 poles (31.1801, -4.1695) (31.2298, -4.2042) (31.3292, -4.2736) (31.4646, -4.3951) (31.5931, -4.5235) (31.7546, -4.7042) (31.9403, -4.9437) (32.1401, -5.2476) (32.3188, -5.5642) (32.4775, -5.8912) (32.6189, -6.2261) (32.6981, -6.4551) (32.7377, -6.5696) knots 0 0 0 0 0.062477 0.124976 0.18748 0.249986 0.374973 0.499971 0.624974 0.749982 0.874991 1 1 1 1 construction
  arc A16 (32.0469, -7.5204) -> (32.7377, -6.5696) centre (22.6957, 0) ccw construction
  spline S33 degree 3 poles (32.0469, -7.5204) (31.9258, -7.5181) (31.6835, -7.5136) (31.3213, -7.4825) (30.9612, -7.4327) (30.6049, -7.3605) (30.2542, -7.2645) (29.969, -7.1618) (29.7473, -7.0641) (29.5854, -6.9815) (29.428, -6.8903) (29.3313, -6.8172) (29.283, -6.7807) knots 0 0 0 0 0.125009 0.250018 0.375026 0.500029 0.625027 0.750014 0.81252 0.875024 0.937523 1 1 1 1 construction
  spline S34 degree 3 poles (29.283, -6.7807) (29.2525, -6.7354) (29.1914, -6.6448) (29.0917, -6.5145) (28.985, -6.39) (28.8689, -6.2743) (28.7485, -6.1629) (28.6168, -6.0649) (28.4789, -5.9762) (28.3325, -5.9017) (28.1787, -5.8443) (28.0192, -5.8052) (27.8557, -5.7878) (27.6916, -5.7958) (27.5301, -5.8269) (27.4022, -5.876) (27.3044, -5.925) (27.2136, -5.9861) (27.1047, -6.0685) (26.9927, -6.1466) (26.9065, -6.214) (26.8298, -6.2919) (26.7436, -6.3984) (26.6641, -6.5424) (26.6057, -6.696) (26.5718, -6.8568) (26.5597, -7.0206) (26.5667, -7.1847) (26.5923, -7.3469) (26.6341, -7.5055) (26.6866, -7.6609) (26.7553, -7.8099) (26.8294, -7.9561) (26.9149, -8.0961) (27.008, -8.2311) (27.0753, -8.3172) (27.1089, -8.3602) knots -0.524268 -0.524268 -0.524268 -0.524268 -0.507879 -0.49149 -0.475102 -0.458716 -0.44233 -0.425942 -0.409559 -0.393171 -0.376784 -0.360403 -0.344025 -0.327651 -0.311278 -0.294912 -0.286715 -0.278522 -0.262134 -0.245745 -0.237552 -0.229355 -0.21299 -0.196616 -0.180243 -0.163864 -0.147483 -0.131097 -0.114709 -0.098325 -0.081938 -0.065552 -0.049165 -0.032777 -0.016389 0 0 0 0 construction
  arc A17 (18.4331, -11.2174) -> (19.5508, -11.5806) centre (22.6957, 0) ccw construction
  spline S35 degree 3 poles (24.0394, -9.3576) (24.0413, -9.303) (24.0451, -9.1938) (24.041, -9.0299) (24.028, -8.8664) (24.002, -8.7045) (23.97, -8.5436) (23.9211, -8.3869) (23.8617, -8.2341) (23.7871, -8.0878) (23.6963, -7.951) (23.5903, -7.8256) (23.4682, -7.7154) (23.3308, -7.6254) (23.1818, -7.5557) (23.0495, -7.5202) (22.9416, -7.5023) (22.8322, -7.4984) (22.6957, -7.5011) (22.5592, -7.4984) (22.4498, -7.5023) (22.3419, -7.5202) (22.2096, -7.5557) (22.0607, -7.6254) (21.9232, -7.7154) (21.8012, -7.8256) (21.6951, -7.951) (21.6044, -8.0878) (21.5297, -8.2341) (21.4703, -8.3869) (21.4214, -8.5436) (21.3895, -8.7045) (21.3635, -8.8664) (21.3504, -9.0299) (21.3463, -9.1938) (21.3501, -9.303) (21.3521, -9.3576) knots -0.524268 -0.524268 -0.524268 -0.524268 -0.507879 -0.49149 -0.475102 -0.458716 -0.44233 -0.425942 -0.409559 -0.393171 -0.376784 -0.360403 -0.344025 -0.327651 -0.311278 -0.294912 -0.286715 -0.278522 -0.262134 -0.245745 -0.237552 -0.229355 -0.21299 -0.196616 -0.180243 -0.163864 -0.147483 -0.131097 -0.114709 -0.098325 -0.081938 -0.065552 -0.049165 -0.032777 -0.016389 0 0 0 0 construction
  circle A18 centre (20.8497, 0) radius 12 construction
  line L29 (64.2812, -31.0434) -> (7.0933, -31.0434)
  line L30 (7.0933, -31.0434) -> (7.0933, 22)
  line L31 (7.0933, 22) -> (64.2812, 22)
  line L32 (64.2812, 22) -> (64.2812, -31.0434)
  circle A19 centre (59.2812, 17) radius 1.4
  circle A20 centre (12.0932, 17) radius 1.4
  circle A21 centre (59.2812, -26.043) radius 1.4
  circle A22 centre (12.0932, -26.043) radius 1.4
  line L33 (64.2812, -304.8) -> (64.2812, 304.8)
  line L34 (7.0933, 304.8) -> (64.2812, 304.8)
  line L35 (7.0933, -304.8) -> (7.0933, 304.8)
  line L36 (64.2812, -304.8) -> (7.0933, -304.8)
  spline S36 degree 3 poles (18.4331, -11.2174) (18.3978, -11.1015) (18.3273, -10.8697) (18.2449, -10.5156) (18.181, -10.1578) (18.1395, -9.7966) (18.1225, -9.4334) (18.132, -9.1304) (18.1564, -8.8894) (18.1849, -8.7099) (18.2231, -8.532) (18.2627, -8.4175) (18.2825, -8.3602) knots 0 0 0 0 0.125009 0.250018 0.375026 0.500029 0.625027 0.750014 0.81252 0.875024 0.937523 1 1 1 1
  spline S37 degree 3 poles (27.1089, -8.3602) (27.1287, -8.4175) (27.1684, -8.532) (27.2065, -8.7099) (27.235, -8.8894) (27.2594, -9.1304) (27.2689, -9.4334) (27.2519, -9.7966) (27.2104, -10.1578) (27.1466, -10.5156) (27.0642, -10.8697) (26.9936, -11.1015) (26.9583, -11.2174) knots 0 0 0 0 0.062477 0.124976 0.18748 0.249986 0.374973 0.499971 0.624974 0.749982 0.874991 1 1 1 1
  spline S38 degree 3 poles (25.8406, -11.5806) (25.744, -11.5076) (25.5507, -11.3615) (25.2758, -11.1235) (25.0139, -10.8715) (24.768, -10.6037) (24.5407, -10.3199) (24.3703, -10.0692) (24.2484, -9.8598) (24.166, -9.6979) (24.0923, -9.5315) (24.057, -9.4156) (24.0394, -9.3576) knots 0 0 0 0 0.125009 0.250018 0.375026 0.500029 0.625027 0.750014 0.81252 0.875024 0.937523 1 1 1 1
  spline S39 degree 3 poles (21.3521, -9.3576) (21.3344, -9.4156) (21.2992, -9.5315) (21.2255, -9.6979) (21.143, -9.8598) (21.0211, -10.0692) (20.8507, -10.3199) (20.6235, -10.6037) (20.3776, -10.8715) (20.1156, -11.1235) (19.8408, -11.3615) (19.6475, -11.5076) (19.5508, -11.5806) knots 0 0 0 0 0.062477 0.124976 0.18748 0.249986 0.374973 0.499971 0.624974 0.749982 0.874991 1 1 1 1
  arc A23 (25.8406, -11.5806) -> (26.9583, -11.2174) centre (22.6957, 0) ccw
  point P0 (64.2812, 0)
  dimension "d0" = 10.15
  dimension "d1" = 22
  dimension "d2" = 5
  dimension "d3" = 5
  dimension "d4" = 2.8
  dimension "d7" = 47.188
  dimension "d10" = 43.043
  dimension "d18" = 0
  constraints: 8 end point, 5 centre point, 3 equal radius, 2 horizontal, 2 parallel, 2 vertical alignment, 1 perpendicular, 6 other
  measures "d0" distance between parallel lines of L29 L10
  measures "d1" distance from line of L31 A18.centre
  measures "d2" distance from line of L31 A19.centre
  measures "d3" distance from line of L32 A19.centre
  measures "d4" diameter of A19
  measures "d7" distance of A19.centre A20.centre
  measures "d10" distance of A19.centre A21.centre
  measures "d18" distance between parallel lines of L35 L30
extrude "Extrusion1" add sketch "Sketch1" against normal blind 21.749 contours L29 L30 L31 L32
sketch "Sketch2" plane through (-57.1879, -22, 0) normal (0, -1, 0) x (1, 0, 0)
  line L0 (57.1879, 18) -> (47.2844, 18) projected
  line L1 (47.2844, 18) -> (47.2844, 17.1148) projected
  spline S0 degree 4 poles (47.2844, 17.1148) (44.146, 16.8158) (35.9341, 19.0327) (29.3273, 12.654) (23.9294, 13.9683) (22.3263, 14.2455) knots 0 0 0 0 0 0.558486 0.866888 0.866888 0.866888 0.866888 0.866888 projected
  line L2 (22.3263, 14.2455) -> (19.9726, 14.071) projected
  line L3 (19.9726, 14.071) -> (19.9726, 13.0329) projected
  line L4 (19.9726, 13.0329) -> (16.0672, 12.6365) projected
  spline S1 degree 2 poles (16.0672, 12.6365) (11.5526, 13.8727) (7.0404, 12.3323) knots 0 0 0 1 1 1 projected
  spline S2 degree 2 poles (7.0404, 12.3323) (3.9856, 12.9721) (0, 11.8599) knots 0 0 0 1 1 1 projected
  line L5 (0, 11.8599) -> (0, 0) projected
  line L6 (0, 0) -> (57.1879, 0) projected
  line L7 (57.1879, 0) -> (57.1879, 18) projected
extrude "Extrusion2" cut sketch "Sketch2" against normal through all
fillet "Fillet1" radius 2.5 4 edges at (-57.1879, -22, 16.8044) (0, -22, 19.8745) (-57.1879, 31.0434, 16.8044) (0, 31.0434, 19.8745)
sketch "Sketch3" plane through (-64.2812, 0, 21.749) normal (0, 0, 1) x (1, 0, 0)
  circle A0 centre (44.6872, -5) radius 1 construction
  circle A1 centre (26.6873, -5) radius 1 construction
  circle A2 centre (26.6873, -5) radius 1.5
  circle A3 centre (44.6872, -5) radius 1.5
  point P0 (64.2812, 0)
  dimension "d23" = 0.5
  dimension "d24" = 0.5
  constraints: 2 centre point
  measures "d23" radial gap between concentric circles of A1 A2
  measures "d24" radial gap between concentric circles of A0 A3
extrude "Extrusion3" cut sketch "Sketch3" against normal blind 67.251
body "Solid1"
